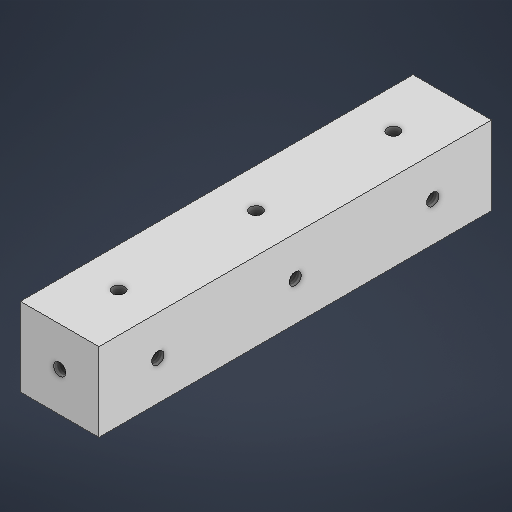
# Autodesk Inventor part: CH3-DiffBoxGussetBlock
Saved by Autodesk Inventor 2026.1 (Build 301233020, 233B)
## iProperties
Created: 2025-10-09
Part Number: CH3-DiffBoxGussetBlock
Material: Generic
Document SubType Name: Modeling
Designer: johnh
Density: 1 g/cm^3
Appearance: Default
Author: johnh
Autodesk Inventor part; units mm, degrees
ref_plane "YZ Plane" through (0, 0, 0) normal (1, 0, 0) x (0, 1, 0)
ref_plane "XZ Plane" through (0, 0, 0) normal (0, 1, 0) x (-1, 0, 0)
ref_plane "XY Plane" through (0, 0, 0) normal (0, 0, 1) x (1, 0, 0)
sketch "Sketch1" plane through (0, 0, 0) normal (0, 0, 1) x (1, 0, 0)
  line L0 (-12.7, -12.7) -> (12.7, -12.7)
  line L1 (12.7, -12.7) -> (12.7, 12.7)
  line L2 (12.7, 12.7) -> (-12.7, 12.7)
  line L3 (-12.7, 12.7) -> (-12.7, -12.7)
  line L4 (-12.7, -12.7) -> (12.7, 12.7) construction
  line L5 (12.7, -12.7) -> (-12.7, 12.7) construction
  point P0 (0, 0)
  dimension "d0" = 25.4
  dimension "d1" = 25.4
  constraints: 12 end point, 2 midpoint, 2 parallel, 1 horizontal, 1 perpendicular
  measures "d0" distance of L1.end L2.end
  measures "d1" distance of L0.end L1.end
extrude "Extrusion1" add sketch "Sketch1" along normal blind 127
sketch "Sketch2" plane through (12.7, -12.7, 0) normal (1, 0, 0) x (0, 0, -1)
  line L0 (-127, 0) -> (-127, 25.4) projected
  line L1 (0, 0) -> (0, 25.4) projected
  line L2 (0, 0) -> (-127, 0) projected
  point P0 (0, 12.7)
  point P1 (-107.95, 12.7)
  point P2 (-63.5, 12.7)
  point P3 (-19.05, 12.7)
  dimension "d4" = 19.05
  dimension "d5" = 127
  dimension "d6" = 63.5
  dimension "d7" = 19.05
  dimension "d27" = 25.4
  dimension "d28" = 12.7
  constraints: 2 horizontal alignment
  measures "d4" distance from line of point (-107.95, 12.7) L0
  measures "d5" distance between parallel lines of L1 L0
  measures "d6" distance from line of point (-63.5, 12.7) L0
  measures "d7" distance from line of point (-19.05, 12.7) L1
  measures "d27" distance of L0.start L0.end
  measures "d28" distance from line of point (-107.95, 12.7) L2
hole "Hole1" at (12.7, 0, 107.95) at (12.7, 0, 63.5) at (12.7, 0, 19.05) direction (-1, 0, 0) diameter 3.9624 depth 12.7 tip angle 118 thread size "10-32 UNF" class "2B" standard "ANSI Unified Screw Threads"
sketch "Sketch3" plane through (-12.7, 12.7, 0) normal (0, 1, 0) x (1, 0, 0)
  line L0 (12.7, -21.0312) -> (12.7, -17.0688) projected
  line L1 (12.7, -65.4812) -> (12.7, -61.5188) projected
  line L2 (12.7, -109.9312) -> (12.7, -105.9688) projected
  line L3 (25.4, -127) -> (0, -127) projected
  line L4 (25.4, 0) -> (0, 0) projected
  line L5 (0, 0) -> (0, -127) projected
  point P0 (12.7, 0)
  point P1 (12.7, -19.05)
  point P2 (12.7, -63.5)
  point P3 (12.7, -107.95)
  constraints: 3 midpoint
hole "Hole2" at (0, 12.7, 19.05) at (0, 12.7, 63.5) at (0, 12.7, 107.95) direction (0, -1, 0) diameter 3.9624 depth 12.7 tip angle 118 thread size "10-32 UNF" class "2B" standard "ANSI Unified Screw Threads"
sketch "Sketch4" plane through (0, 0, 127) normal (0, 0, 1) x (1, 0, 0)
  point P0 (0, 0)
  point P1 (0, 0)
  constraints: 1 coincident
hole "Hole3" at (0, 0, 127) direction (0, 0, -1) diameter 3.9624 depth 25.4 tip angle 118 thread size "10-32 UNF" class "2B" standard "ANSI Unified Screw Threads"
sketch "Sketch5" plane through (0, 0, 0) normal (0, 0, -1) x (-1, 0, 0)
  point P0 (0, 0)
  point P1 (0, 0)
  constraints: 1 coincident
hole "Hole4" at (0, 0, 0) direction (0, 0, 1) diameter 3.9624 depth 25.4 tip angle 118 thread size "10-32 UNF" class "2B" standard "ANSI Unified Screw Threads"
equation "\"d6\" = 0.5 * d5"
equation "\"d7\" = d4"
equation "\"d28\" = 0.5 * d27"
body "Solid1"
